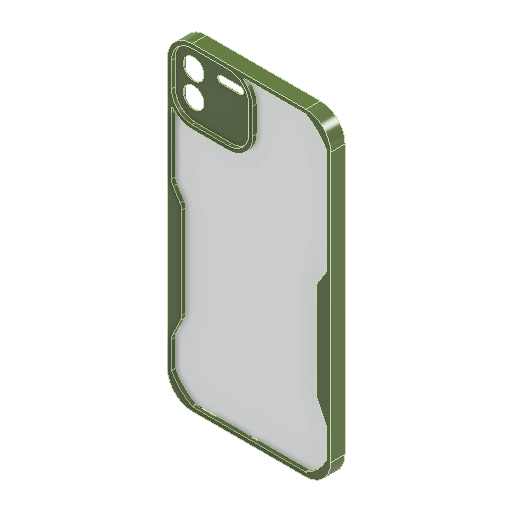
# Autodesk Inventor part: prashantPhone
Saved by Autodesk Inventor 2025.2 (Build 292293000, 293)
## iProperties
Created: 2025-05-30
Part Number: prashantPhone
Material: Glass
Document SubType Name: Modeling
Designer: spars
Density: 2.18 g/cm^3
Appearance: Dark Olive
Author: spars
Autodesk Inventor part; units mm, degrees
ref_plane "YZ Plane" through (0, 0, 0) normal (1, 0, 0) x (0, 1, 0)
ref_plane "XZ Plane" through (0, 0, 0) normal (0, 1, 0) x (-1, 0, 0)
sketch "Sketch1" plane through (0, 0, 0) normal (0, 0, 1) x (1, 0, 0)
  line L0 (-27.2929, -75) -> (27.5, -75)
  line L1 (37.5, -65) -> (37.5, 64.7929)
  line L2 (-37.5, 53) -> (-37.5, -64.7929)
  line L3 (-27.5, 75) -> (-10, 75)
  line L4 (0, 65) -> (0, 53)
  line L5 (-10, 43) -> (-27.5, 43)
  line L6 (-37.5, 53) -> (-37.5, 65)
  circle A0 centre (-28.5, 65) radius 5
  circle A1 centre (-28.5, 53) radius 5
  line L7 (-15.2122, 67.2387) -> (-5.9397, 67.2387) construction
  line L8 (-15.2122, 65.5268) -> (-5.9397, 65.5268)
  line L9 (-5.9397, 68.9505) -> (-15.2122, 68.9505)
  arc A2 (-15.2122, 68.9505) -> (-15.2122, 65.5268) centre (-15.2122, 67.2387) ccw
  arc A3 (-5.9397, 65.5268) -> (-5.9397, 68.9505) centre (-5.9397, 67.2387) ccw
  arc A4 (-10, 43) -> (0, 53) centre (-10, 53) ccw
  arc A5 (0, 65) -> (-10, 75) centre (-10, 65) ccw
  arc A6 (-37.5, 53) -> (-27.5, 43) centre (-27.5, 53) ccw
  arc A7 (-27.5, 75) -> (-37.5, 65) centre (-27.5, 65) ccw
  line L10 (-27.5, 43) -> (-37.5, 43)
  arc A8 (37.5, 65) -> (27.5, 75) centre (27.5, 65) ccw
  arc A9 (-37.5, -65) -> (-27.5, -75) centre (-27.5, -65) ccw
  arc A10 (27.5, -75) -> (37.5, -65) centre (27.5, -65) ccw
  arc A11 (-27.5, 75) -> (-37.5, 65) centre (-27.5, 65) ccw
  line L11 (-36.7048, 12.652) -> (-33.2952, 7.3532)
  line L12 (-32.5, 4.6477) -> (-32.5, -39.3494)
  line L13 (-33.0083, -41.5459) -> (-36.9917, -49.6915)
  arc A12 (-32.5, 4.6477) -> (-33.2952, 7.3532) centre (-37.5, 4.6477) ccw
  arc A13 (-36.9917, -49.6915) -> (-37.5, -51.8881) centre (-32.5, -51.8881) ccw
  arc A14 (-37.5, 15.3576) -> (-36.7048, 12.652) centre (-32.5, 15.3576) ccw
  line L14 (36.7048, 12.652) -> (33.2952, 7.3532)
  line L15 (32.5, 4.6477) -> (32.5, -40.5065)
  line L16 (32.5, -40.5065) -> (36.9917, -49.6915)
  arc A15 (33.2952, 7.3532) -> (32.5, 4.6477) centre (37.5, 4.6477) ccw
  arc A16 (37.5, -51.8881) -> (36.9917, -49.6915) centre (32.5, -51.8881) ccw
  arc A17 (36.7048, 12.652) -> (37.5, 15.3576) centre (32.5, 15.3576) ccw
  arc A18 (-33.0083, -41.5459) -> (-32.5, -39.3494) centre (-37.5, -39.3494) ccw
  arc A19 (-27.5, 77) -> (-39.5, 65) centre (-27.5, 65) ccw
  line L17 (-27.5, 77) -> (27.5, 77)
  arc A20 (39.5, 65) -> (27.5, 77) centre (27.5, 65) ccw
  line L18 (39.5, 65) -> (39.5, -65)
  arc A21 (27.5, -77) -> (39.5, -65) centre (27.5, -65) ccw
  line L19 (27.5, -77) -> (-27.5, -77)
  arc A22 (-39.5, -65) -> (-27.5, -77) centre (-27.5, -65) ccw
  line L20 (-39.5, -65) -> (-39.5, 53)
  line L21 (-39.5, 65) -> (-39.5, 53)
  arc A23 (-36.6173, 45.3354) -> (-27.5, 41.089) centre (-27.5, 53) ccw
  line L22 (-27.5, 41.089) -> (-10, 41.089)
  arc A24 (-10, 41.089) -> (1.911, 53) centre (-10, 53) ccw
  line L23 (1.911, 53) -> (1.911, 65.5801)
  arc A25 (1.911, 65.5801) -> (-2.314, 74.1177) centre (-10, 65) ccw
  line L24 (-10, 76.9251) -> (-27.5, 76.9251)
  arc A26 (-27.5, 76.9251) -> (-39.4251, 65) centre (-27.5, 65) ccw
  line L25 (-39.4251, 65) -> (-39.4251, 53)
  arc A27 (-36.6173, 45.3354) -> (-37.5, 45.0136) centre (-37, 45.0136) ccw
  line L26 (27.5, 75) -> (-10, 75)
  line L27 (-10, 75) -> (-27.5, 75)
  arc A28 (-1.9917, 75) -> (-2.314, 74.1177) centre (-1.9917, 74.5) ccw
  line L28 (-37.5, -56.9135) -> (-37.5, -65)
  line L29 (-27.5, -75) -> (-19.6948, -75)
  arc A29 (-37.5, -64.7929) -> (-37.4435, -65.0238) centre (-37, -64.7929) ccw
  arc A30 (-27.5238, -74.9435) -> (-27.2929, -75) centre (-27.2929, -74.5) ccw
  arc A31 (-37.4435, -65.0238) -> (-27.5238, -74.9435) centre (-16.7467, -54.2467) ccw
  arc A32 (37.4435, -65.0238) -> (37.5, -64.7929) centre (37, -64.7929) ccw
  arc A33 (27.2929, -75) -> (27.5238, -74.9435) centre (27.2929, -74.5) ccw
  arc A34 (27.5238, -74.9435) -> (37.4435, -65.0238) centre (16.7467, -54.2467) ccw
  line L30 (27.2929, 75) -> (17.9376, 75)
  line L31 (37.5, 65) -> (37.5, 56.6526)
  arc A35 (27.5419, 74.9336) -> (27.2929, 75) centre (27.2929, 74.5) ccw
  arc A36 (37.5, 64.7929) -> (37.4336, 65.0419) centre (37, 64.7929) ccw
  arc A37 (37.4336, 65.0419) -> (27.5419, 74.9336) centre (14.1903, 51.6903) ccw
  point P0 (0, 0)
  point P1 (0, 43)
  point P2 (-10.576, 67.2387)
  point P3 (-37.5, 13.8879)
  point P4 (-32.5, -40.5065)
  point P5 (-37.5, 46.5292)
  point P6 (-3.5033, 75)
  point P7 (-37.5, 65)
  point P8 (37.5, 15.3576)
  point P9 (-33.9708, 43)
  dimension "d3" = 10
  dimension "d4" = 10
  dimension "d6" = 10
  dimension "d9" = 10
  dimension "d10" = 10
  dimension "d12" = 5
  dimension "d13" = 5
  dimension "d14" = 5
  dimension "d15" = 2
  dimension "d16" = 0.5
  dimension "d17" = 0.5
  dimension "d18" = 0.5
  dimension "d19" = 0.5
  constraints: 75 point on circle, 64 end point, 38 centre point, 37 tangent, 13 point on line, 9 equal radius, 7 parallel, 4 horizontal, 4 vertical, 3 perpendicular, 1 midpoint, 26 other
  measures "d3" diameter of A0
  measures "d4" diameter of A1
  measures "d6" distance from line of L5 A1.centre
  measures "d9" radius of A4
  measures "d10" radius of A8
  measures "d12" radius of A12
  measures "d13" radius of A14
  measures "d14" radius of A18
  measures "d15" distance between parallel lines of L0 L19
  measures "d16" radius of A27
  measures "d17" radius of A28
  measures "d18" radius of A29
  measures "d19" radius of A35
extrude "Extrusion1" add sketch "Sketch1" along normal blind 2 and the other way blind 5 contours L17 A20 L18 A21 L19 A22 L20 L21 A19
extrude "Extrusion2" add sketch "Sketch1" along normal blind 2 contours L29 A9 L28 A29 A31 A30 | A33 A34 A32 L1 A10 L0 | L2 A14 L11 A12 L12 A18 L13 A13 | A16 L16 L15 A15 L14 A17 L1 | A36 A37 A35 L26 A8 L31
extrude "Extrusion3" add sketch "Sketch1" along normal blind 2 contours L2 A6 L10 A23 A27 | L10 L5 A4 L4 A5 L26 A28 A25 L23 A24 L22 A23
extrude "Extrusion4" add sketch "Sketch1" along normal mid plane 0.5 contours L6 A7 L3 A5 L4 A4 L5 A6
extrude "Extrusion5" add sketch "Sketch1" against normal blind 1 contours A30 A31 A29 L2 A13 L13 A18 L12 A12 L11 A14 L10 A23 L22 A24 L23 A25 A28 L26 A35 A37 A36 L1 A17 L14 A15 L15 L16 A16 A32 A34 A33 L0 | L29 A9 L28 A29 A31 A30 | A33 A34 A32 L1 A10 L0 | L2 A14 L11 A12 L12 A18 L13 A13 | A16 L16 L15 A15 L14 A17 L1 | A36 A37 A35 L26 A8 L31
sketch "Sketch2" plane through (0, 0, -1) normal (0, 0, -1) x (-1, 0, 0)
  arc A0 (33.9708, 43) -> (36.6173, 45.3354) centre (27.5, 53) ccw projected
  arc A1 (37.5, 45.0136) -> (36.6173, 45.3354) centre (37, 45.0136) ccw projected
  line L0 (37.5, 43) -> (33.9708, 43) projected
  line L1 (37.5, 65) -> (37.5, -65) projected
  point P0 (0, 0)
extrude "Extrusion6" add sketch "Sketch2" against normal blind 2
sketch "Sketch3" plane through (-39.5, -65, 2) normal (-1, 0, 0) x (0, 0, 1)
  line L0 (-3.6421, 4.5891) -> (-3.6421, 15.3057) construction
  line L1 (-2, 0.2071) -> (-2, 13.1119) projected
  line L2 (-1.5535, 4.5891) -> (-1.5535, 15.3057)
  line L3 (-5.7306, 15.3057) -> (-5.7306, 4.5891)
  arc A0 (-5.7306, 4.5891) -> (-1.5535, 4.5891) centre (-3.6421, 4.5891) ccw
  arc A1 (-1.5535, 15.3057) -> (-5.7306, 15.3057) centre (-3.6421, 15.3057) ccw
  circle A2 centre (-3.6421, 15.3057) radius 1.012
  circle A3 centre (-3.6421, 4.5891) radius 1.012
  line L4 (-3.6421, 100.347) -> (-3.6421, 108.9069) construction
  line L5 (-2, 129.7929) -> (-2, 80.3576) projected
  line L6 (-1.5535, 100.347) -> (-1.5535, 108.9069)
  line L7 (-5.7306, 108.9069) -> (-5.7306, 100.347)
  arc A4 (-5.7306, 100.347) -> (-1.5535, 100.347) centre (-3.6421, 100.347) ccw
  arc A5 (-1.5535, 108.9069) -> (-5.7306, 108.9069) centre (-3.6421, 108.9069) ccw
  line L8 (-3.6421, 113.6704) -> (-3.6421, 119.2482) construction
  line L9 (-1.5312, 113.6704) -> (-1.5312, 119.2482)
  line L10 (-5.753, 119.2482) -> (-5.753, 113.6704)
  arc A6 (-5.753, 113.6704) -> (-1.5312, 113.6704) centre (-3.6421, 113.6704) ccw
  arc A7 (-1.5312, 119.2482) -> (-5.753, 119.2482) centre (-3.6421, 119.2482) ccw
  line L11 (-5.9747, 100.347) -> (-5.9747, 108.9069)
  arc A8 (-1.3094, 108.9069) -> (-5.9747, 108.9069) centre (-3.6421, 108.9069) ccw
  line L12 (-1.3094, 108.9069) -> (-1.3094, 100.347)
  arc A9 (-5.9747, 100.347) -> (-1.3094, 100.347) centre (-3.6421, 100.347) ccw
  line L13 (-5.0322, 113.6704) -> (-5.0322, 119.2482)
  arc A10 (-2.2519, 119.2482) -> (-5.0322, 119.2482) centre (-3.6421, 119.2482) ccw
  line L14 (-2.2519, 119.2482) -> (-2.2519, 113.6704)
  arc A11 (-5.0322, 113.6704) -> (-2.2519, 113.6704) centre (-3.6421, 113.6704) ccw
  point P0 (-2, 65)
  point P1 (-3.6421, 9.9474)
  point P2 (-3.6421, 104.627)
  point P3 (-3.6421, 116.4593)
  constraints: 32 end point, 20 point on circle, 12 centre point, 12 tangent, 7 parallel, 3 midpoint, 2 point on line, 6 other
extrude "Extrusion7" cut sketch "Sketch3" against normal blind 2 contours A2 | A3
extrude "Extrusion8" cut sketch "Sketch3" against normal blind 0.2 contours A0 L3 A1 L2
extrude "Extrusion9" add sketch "Sketch3" along normal blind 0.2 contours A5 L6 A4 L5 | L5 A4 L7 A5
extrude "Extrusion10" cut sketch "Sketch3" against normal blind 0.2 contours A8 L12 A9 L5 A4 L6 A5 | L5 A5 L7 A4 A9 L11 A8
extrude "Extrusion11" add sketch "Sketch3" along normal blind 0.2 contours L13 A10 L14 A11
extrude "Extrusion12" cut sketch "Sketch3" against normal blind 0.2 contours A7 L9 A6 L5 | L5 A6 L10 A7
sketch "Sketch4" plane through (-39.5, -65, 2) normal (-1, 0, 0) x (0, 0, 1)
  line L0 (-5.9747, 100.347) -> (-5.9747, 108.9069) projected
  line L1 (-5.7306, 108.9069) -> (-5.7306, 100.347) projected
  arc A0 (-1.3094, 108.9069) -> (-5.9747, 108.9069) centre (-3.6421, 108.9069) ccw projected
  arc A1 (-1.5535, 108.9069) -> (-5.7306, 108.9069) centre (-3.6421, 108.9069) ccw projected
  line L2 (-1.5535, 100.347) -> (-1.5535, 108.9069) projected
  arc A2 (-5.7306, 100.347) -> (-1.5535, 100.347) centre (-3.6421, 100.347) ccw projected
  arc A3 (-5.9747, 100.347) -> (-1.3094, 100.347) centre (-3.6421, 100.347) ccw projected
  line L3 (-1.3094, 108.9069) -> (-1.3094, 100.347) projected
  line L4 (-1.5312, 119.2482) -> (-1.5312, 113.6704) projected
  arc A4 (-5.753, 113.6704) -> (-1.5312, 113.6704) centre (-3.6421, 113.6704) ccw projected
  line L5 (-5.753, 113.6704) -> (-5.753, 119.2482) projected
  arc A5 (-1.5312, 119.2482) -> (-5.753, 119.2482) centre (-3.6421, 119.2482) ccw projected
  arc A6 (-1.3094, 108.9069) -> (-5.9747, 108.9069) centre (-3.6421, 108.9069) ccw projected
  line L6 (-1.3094, 108.9069) -> (-1.3094, 100.347) projected
  arc A7 (-5.9747, 100.347) -> (-1.3094, 100.347) centre (-3.6421, 100.347) ccw projected
  line L7 (-5.9747, 100.347) -> (-5.9747, 108.9069) projected
  line L8 (-1.5535, 15.3057) -> (-1.5535, 4.5891) projected
  arc A8 (-5.7306, 4.5891) -> (-1.5535, 4.5891) centre (-3.6421, 4.5891) ccw projected
  line L9 (-5.7306, 4.5891) -> (-5.7306, 15.3057) projected
  arc A9 (-1.5535, 15.3057) -> (-5.7306, 15.3057) centre (-3.6421, 15.3057) ccw projected
  line L10 (-7, 0) -> (0, 0) projected
  line L11 (0, 130) -> (0, 0) projected
  line L12 (-7, 130) -> (0, 130) projected
  line L13 (-7, 0) -> (-7, 130) projected
  line L14 (-5.0322, 119.2482) -> (-5.0322, 113.6704) projected
  arc A10 (-5.0322, 113.6704) -> (-2.2519, 113.6704) centre (-3.6421, 113.6704) ccw projected
  line L15 (-5.0322, 119.2482) -> (-5.0322, 113.6704) projected
  arc A11 (-5.0322, 113.6704) -> (-2.2519, 113.6704) centre (-3.6421, 113.6704) ccw projected
  line L16 (-2.2519, 113.6704) -> (-2.2519, 119.2482) projected
  arc A12 (-2.2519, 119.2482) -> (-5.0322, 119.2482) centre (-3.6421, 119.2482) ccw projected
  point P0 (-2, 65)
sketch "Sketch5" plane through (-37.5, -65, -5) normal (1, 0, 0) x (0, 0, -1)
  point P0 (-5, 65)
ref_plane "Work Plane2" through (-37.5, -65, -5) normal (1, 0, 0) x (0, 0, -1)
ref_plane "Work Plane1" through (-38.5, -65, -5) normal (1, 0, 0) x (0, 0, -1)
sketch "Sketch7" plane through (-27.5, -77, 2) normal (0, -1, 0) x (1, 0, 0)
  line L0 (25.0083, 0) -> (25.0083, -2) projected
  line L1 (29.9917, -5.0839) -> (25.0083, -5.0839)
  line L2 (25.0083, -5.0839) -> (25.0083, -1.5482)
  line L3 (25.0083, -1.5482) -> (29.9917, -1.5482)
  line L4 (29.9917, -1.5482) -> (29.9917, -5.0839)
  line L5 (0, -3) -> (55, -3) projected
  line L6 (10.5634, -3) -> (0.4234, -3) construction
  line L7 (9.0799, -1.5165) -> (1.9069, -1.5165)
  line L8 (1.9069, -4.4835) -> (9.0799, -4.4835)
  arc A0 (9.0799, -4.4835) -> (9.0799, -1.5165) centre (9.0799, -3) ccw
  arc A1 (1.9069, -1.5165) -> (1.9069, -4.4835) centre (1.9069, -3) ccw
  line L9 (0, -7) -> (0, 0) projected
  line L10 (55, -7) -> (55, 0) projected
  line L11 (55, -7) -> (0, -7) projected
  point P0 (27.5, -2)
  point P1 (5.4934, -3)
  point P2 (27.5, -5.0839)
  dimension "d47" = 55
  dimension "d48" = 27.5
  dimension "d49" = 27.5
  dimension "d50" = 2.5165
  constraints: 16 end point, 6 point on circle, 5 point on line, 4 tangent, 3 parallel, 2 centre point, 2 midpoint, 1 horizontal, 1 perpendicular
  measures "d47" distance between parallel lines of L9 L10
  measures "d48" distance from line of point (27.5, -5.084) L10
  measures "d49" distance from line of L9 point (27.5, -5.084)
  measures "d50" distance between parallel lines of L11 L8
extrude "Extrusion13" cut sketch "Sketch7" against normal blind 2 contours L3 L4 L5 L2 L0 | L5 L4 L1 L2 | A0 L8 A1 L5 | L5 A1 L7 A0
body "Solid1"
